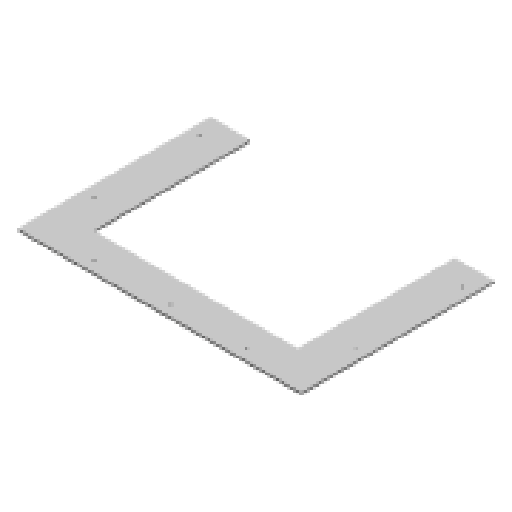
# Autodesk Inventor part: TopBrace
Saved by Autodesk Inventor 2023.2 (Build 272271000, 271)
## iProperties
Created: 2022-04-12
Part Number: TopBrace
Material: Aluminum 6061
Document SubType Name: Modeling
Designer: Remo
Density: 2.7 g/cm^3
Appearance: Anodized - Light Gray
Author: Remo
Autodesk Inventor part; units mm, degrees
ref_plane "YZ Plane" through (0, 0, 0) normal (1, 0, 0) x (0, 1, 0)
ref_plane "XZ Plane" through (0, 0, 0) normal (0, 1, 0) x (-1, 0, 0)
ref_plane "XY Plane" through (0, 0, 0) normal (0, 0, 1) x (1, 0, 0)
sketch "Sketch1" plane through (0, 0, 0) normal (0, 1, 0) x (-1, 0, 0)
  line L0 (-195, -265.5) -> (195, -265.5)
  line L1 (195, -265.5) -> (195, 265.5)
  line L2 (195, 265.5) -> (-195, 265.5)
  line L3 (-195, 265.5) -> (-195, -265.5)
  line L4 (-195, -265.5) -> (195, 265.5) construction
  line L5 (195, -265.5) -> (-195, 265.5) construction
  line L6 (-140, -215.5) -> (140, -215.5)
  line L7 (140, -215.5) -> (140, 215.5)
  line L8 (140, 215.5) -> (-140, 215.5)
  line L9 (-140, 215.5) -> (-140, -215.5)
  line L10 (-140, -215.5) -> (140, 215.5) construction
  line L11 (140, -215.5) -> (-140, 215.5) construction
  line L12 (195, 0) -> (140, 0)
  line L13 (-140, 0) -> (-195, 0)
  circle A0 centre (180, 175.5) radius 1.75
  circle A1 centre (180, 30) radius 1.75
  circle A2 centre (-180, 30) radius 1.75
  circle A3 centre (-180, 175.5) radius 1.75
  circle A4 centre (105, 250.5) radius 1.75
  circle A5 centre (-105, 250.5) radius 1.75
  circle A6 centre (0, 250.5) radius 1.75
  point P0 (0, 0)
  point P1 (167.5, 0)
  point P2 (0, 215.5)
  dimension "d0" = 390
  dimension "d1" = 531
  dimension "d2" = 50
  dimension "d3" = 55
  dimension "d4" = 15
  dimension "d5" = 15
  dimension "d6" = 15
  dimension "d7" = 30
  dimension "d8" = 3.5
  dimension "d9" = 90
  dimension "d10" = 90
  dimension "d11" = 90
  constraints: 28 end point, 10 midpoint, 7 centre point, 6 equal radius, 4 horizontal alignment, 4 parallel, 3 vertical alignment, 2 horizontal, 2 perpendicular
  measures "d0" distance of L1.end L2.end
  measures "d1" distance of L0.end L1.end
  measures "d2" distance between parallel lines of L2 L8
  measures "d3" distance between parallel lines of L1 L7
  measures "d4" distance from line of L1 A0.centre
  measures "d5" distance from line of L3 A3.centre
  measures "d6" distance from line of L2 A4.centre
  measures "d7" vertical distance of point (167.5, 0) A1.centre
  measures "d8" diameter of A1
  measures "d9" distance from line of L2 A0.centre
  measures "d10" distance from line of L1 A4.centre
  measures "d11" distance from line of L3 A5.centre
extrude "Extrusion1" add sketch "Sketch1" along normal blind 3 contours L3 L2 L1 L12 L7 L8 L9 L13
fillet "Fillet1" radius 2 4 edges at (195, 1.5, 265.5) (-195, 1.5, 265.5) (140, 1.5, 215.5) (-140, 1.5, 215.5)
equation "\"d5\" = d4"
equation "\"d6\" = d4"
equation "\"d11\" = d10"
body "Solid1"
